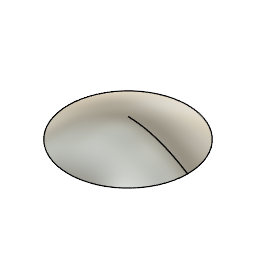
Mouse_Tip_v1 (Autodesk Fusion 360 design; units mm, degrees)
Autodesk Fusion 360 part; units mm, degrees
sketch "Skizze1" plane through (0, 0, 0) normal (0, 1, 0) x (1, 0, 0)
  line L0 (0, 0) -> (6, 0)
  line L1 (0, 0) -> (0, -2)
  spline S0 degree 5 poles (0, -2) (0.24, -2) (0.72, -1.9826) (1.44, -1.9042) (2.4, -1.6981) (3.6, -1.2838) (4.56, -0.8373) (5.28, -0.4418) (5.76, -0.1517) (6, 0) knots 0.5 0.5 0.5 0.5 0.5 0.5 0.6 0.7 0.8 0.9 1 1 1 1 1 1
  line L2 (-0.6245, -2) -> (0.6245, -2)
  constraint coincident L0.start L1.start
  constraint perpendicular L0 L1
  constraint coincident L1 L0.start
  constraint midpoint L1.end L2
revolve "Drehen1" add sketch "Skizze1" angle 360 about axis through (0, 0, 1.75) along (0, 0, 1)
